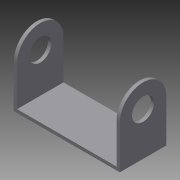
# Autodesk Inventor part: Wrist_Roll
Saved by Autodesk Inventor 2013 (Build 170138000, 138)
## iProperties
Created: 2012-12-04
Part Number: Wrist_Roll
Material: Generic
Document SubType Name: Modeling
Designer: Joe
Density: 1 g/cm^3
Author: Joe
Autodesk Inventor part; units mm, degrees
ref_plane "YZ Plane" through (0, 0, 0) normal (1, 0, 0) x (0, 1, 0)
ref_plane "XZ Plane" through (0, 0, 0) normal (0, 1, 0) x (-1, 0, 0)
ref_plane "XY Plane" through (0, 0, 0) normal (0, 0, 1) x (1, 0, 0)
sketch "Sketch1" plane through (0, 0, 0) normal (0, 0, 1) x (1, 0, 0)
  circle A0 centre (0, 0) radius 10
  arc A1 (21, 0) -> (-21, 0) centre (0, 0) ccw
  line L0 (0, 0) -> (0, -39) construction
  line L1 (0, -39) -> (21, -39)
  line L2 (0, -39) -> (-21, -39)
  line L3 (-21, -39) -> (-21, 0)
  line L4 (21, -39) -> (21, 0)
  dimension "d0" = 20
  dimension "d2" = 42
  dimension "d3" = 21
  dimension "d4" = 39
  constraints: 10 end point, 2 centre point, 2 coincident, 2 collinear, 2 point on circle, 2 tangent, 1 perpendicular, 1 vertical
  measures "d0" diameter of A0
  measures "d2" diameter of A1
  measures "d3" distance of L0.end L1.end
  measures "d4" distance of L0.start L0.end
extrude "Extrusion1" add sketch "Sketch1" along normal mid plane 96
sketch "Sketch2" plane through (0, 0, 0) normal (0, 0, 1) x (1, 0, 0)
  circle A0 centre (0, 0) radius 10 projected
  line L0 (-21, -39) -> (21, -39) projected
  line L1 (21, -39) -> (21, 0) projected
  arc A1 (21, 0) -> (-21, 0) centre (0, 0) ccw projected
  line L2 (-21, 0) -> (-21, -39) projected
  line L3 (-21, -36) -> (21, -36)
  line L4 (21, -36) -> (21, 0)
  line L5 (-21, -31.2069) -> (-21, 0)
  dimension "d7" = 3
  constraints: 6 end point, 3 point on line, 2 perpendicular, 2 tangent, 1 collinear
  measures "d7" distance between parallel lines of L0 L3
extrude "Extrusion2" cut sketch "Sketch2" along normal mid plane 90 contours L2 A1 L1 L3
move or copy body "Move Body1" bodies to move or copy 1 copy no rotation origin (0, 0, 0) rotation axis (1, 0, 0) rotation angle 90
move or copy body "Move Body2" bodies to move or copy 1 copy no rotation origin (0, 0, 0) rotation axis (0, 0, 1) rotation angle 90
body "Solid1"
